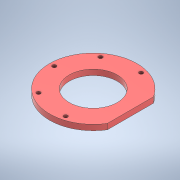
# Autodesk Inventor part: держалка подша
Saved by Autodesk Inventor 2022 (Build 260153000, 153)
## iProperties
Created: 2022-12-27
Part Number: держалка подша
Material: Типовые
Document SubType Name: Modeling
Designer: Pavel
Density: 1 g/cm^3
Appearance: По умолчанию
Author: Pavel
Autodesk Inventor part; units mm, degrees
ref_plane "YZ Plane" through (0, 0, 0) normal (1, 0, 0) x (0, 1, 0)
ref_plane "XZ Plane" through (0, 0, 0) normal (0, 1, 0) x (-1, 0, 0)
ref_plane "XY Plane" through (0, 0, 0) normal (0, 0, 1) x (1, 0, 0)
sketch "Эскиз1" plane through (0, 0, 0) normal (0, 1, 0) x (-1, 0, 0)
  circle A0 centre (0, 0) radius 13
  arc A1 (-20.1, -12.4624) -> (-20.1, 12.4624) centre (0, 0) ccw
  line L0 (-20.1, 12.4624) -> (-20.1, -12.4624)
  line L1 (-20.1, 0) -> (21.15, 0)
  circle A2 centre (21.15, 0) radius 1.05
  circle A3 centre (12.8753, 16.7794) radius 1.05
  circle A4 centre (-5.474, 20.4293) radius 1.05
  circle A5 centre (12.8753, -16.7794) radius 1.05
  circle A6 centre (-5.474, -20.4293) radius 1.05
  dimension "d0" = 26
  dimension "d1" = 47.3
  dimension "d3" = 2.1
  dimension "d4" = 21.15
  dimension "d11" = 20.1
  dimension "d24" = 105
  dimension "d28" = 105
  constraints: 7 centre point, 4 end point, 3 coincident, 2 point on circle, 1 horizontal, 1 midpoint, 1 vertical, 10 other
  measures "d0" diameter of A0
  measures "d1" diameter of A1
  measures "d3" diameter of A2
  measures "d4" distance of L1.end point (0, 0)
  measures "d11" distance from line of L0 point (0, 0)
extrude "Выдавливание3" add sketch "Эскиз1" along normal blind 3
